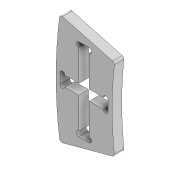
# Autodesk Inventor part: Feet - V2
Saved by Autodesk Inventor 2020 (Build 240168000, 168)
## iProperties
Created: 2020-03-12
Part Number: Feet - V2
Material: Generic
Document SubType Name: Modeling
Designer: Daniel Wikman
Density: 1 g/cm^3
Appearance: Default
Author: Daniel Wikman
Autodesk Inventor part; units mm, degrees
ref_plane "YZ Plane" through (0, 0, 0) normal (1, 0, 0) x (0, 1, 0)
ref_plane "XZ Plane" through (0, 0, 0) normal (0, 1, 0) x (-1, 0, 0)
ref_plane "XY Plane" through (0, 0, 0) normal (0, 0, 1) x (1, 0, 0)
sketch "Sketch1" plane through (0, 0, 0) normal (0, 0, 1) x (1, 0, 0)
  line L0 (-3.75, 30) -> (3.75, 30)
  arc A0 (-14, 3.75) -> (-17.5, 3.75) centre (-15.75, 3.75) ccw
  arc A1 (-3.75, 30) -> (-3.75, 26.5) centre (-3.75, 28.25) ccw
  arc A2 (3.75, 26.5) -> (3.75, 30) centre (3.75, 28.25) ccw
  line L1 (272, 51.0746) -> (272, -58.8764)
  line L2 (-17.5, 0) -> (30.5939, 0)
  line L3 (-17.5, 3.75) -> (-17.5, 0)
  arc A3 (-17.5, -3.75) -> (-14, -3.75) centre (-15.75, -3.75) ccw
  line L4 (-17.5, -3.75) -> (-17.5, 0)
  line L5 (0, 0) -> (0, -60.7814)
  line L6 (-14, 3.75) -> (-3.75, 3.75)
  line L7 (-14, -3.75) -> (-3.75, -3.75)
  line L8 (-3.75, 26.5) -> (-3.75, 3.75)
  line L9 (3.75, 26.5) -> (3.75, 3.75)
  arc A4 (17.5, 3.75) -> (14, 3.75) centre (15.75, 3.75) ccw
  line L10 (17.5, 3.75) -> (17.5, 0)
  line L11 (17.5, -3.75) -> (17.5, 0)
  arc A5 (14, -3.75) -> (17.5, -3.75) centre (15.75, -3.75) ccw
  line L12 (14, 3.75) -> (3.75, 3.75)
  line L13 (14, -3.75) -> (3.75, -3.75)
  line L14 (-3.75, -30) -> (3.75, -30)
  arc A6 (-3.75, -26.5) -> (-3.75, -30) centre (-3.75, -28.25) ccw
  arc A7 (3.75, -30) -> (3.75, -26.5) centre (3.75, -28.25) ccw
  line L15 (3.75, -26.5) -> (3.75, -3.75)
  line L16 (-3.75, -26.5) -> (-3.75, -3.75)
  line L17 (-20.5, 0) -> (-17.5, 0)
  line L18 (17.5, 0) -> (20.5, 0)
  arc A8 (-17.6845, 40.4864) -> (-17.6845, -40.4864) centre (272, 0) ccw
  arc A9 (22.2694, 29.7808) -> (22.2694, -29.7808) centre (272, 0) ccw
  line L19 (22.2694, -29.7808) -> (-17.6845, -40.4864)
  line L20 (22.2694, 29.7808) -> (-17.6845, 40.4864)
  point P0 (-34.7553, 50.5125)
  point P1 (74.6913, 21.1864)
  point P2 (-34.7553, -50.5125)
  point P3 (74.6913, -21.1864)
  dimension "d3" = 1.75
  dimension "d43" = 0
  dimension "d46" = 7.5
  dimension "d47" = 1.75
  dimension "d48" = 1.75
  dimension "d49" = 7.5
  dimension "d50" = 7.5
  dimension "d51" = 60
  dimension "d52" = 35
  dimension "d55" = 3
  dimension "d57" = 585
  dimension "d58" = 3
  dimension "d61" = 15
  constraints: 42 end point, 22 point on circle, 21 symmetric about line, 10 centre point, 4 point on line, 3 horizontal, 3 perpendicular, 2 vertical, 1 coincident, 1 collinear, 5 other
  measures "d3" radius of A0
  measures "d43" distance from line of L5.start L2
  measures "d46" distance of L9.start L8.start
  measures "d47" radius of A2
  measures "d48" radius of A1
  measures "d49" distance of L0.start L0.end
  measures "d50" diameter of L8.start L5
  measures "d51" diameter of L0 L2
  measures "d52" diameter of L3 L5
  measures "d55" distance of L17.start L2.start
  measures "d57" diameter of L17.start L1
  measures "d58" distance of L10.end L18.end
  measures "d61" angle of L2 L19
extrude "Extrusion1" add sketch "Sketch1" along normal blind 7 contours A1 L8 L6 A0 L3 L17 A8 L20 A9 L2 L10 A4 L12 L9 A2 L0 | L4 A3 L7 L16 A6 L14 L5 L19 A8 L17 | L2 A9 L19 L5 L14 A7 L15 L13 A5 L11
fillet "Fillet1" radius 1.75 4 edges at (-17.6845, -40.4864, 3.5) (22.2694, -29.7808, 3.5) (22.2694, 29.7808, 3.5) (-17.6845, 40.4864, 3.5)
body "Solid1"
